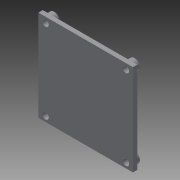
# Autodesk Inventor part: platnickapoddriver
Saved by Autodesk Inventor 2013 (Build 170138000, 138)
## iProperties
Created: 2015-06-20
Part Number: platnickapoddriver
Material: Generic
Document SubType Name: Modeling
Designer: Jufo
Density: 1 g/cm^3
Author: Jufo
Autodesk Inventor part; units mm, degrees
ref_plane "YZ Plane" through (0, 0, 0) normal (1, 0, 0) x (0, 1, 0)
ref_plane "XZ Plane" through (0, 0, 0) normal (0, 1, 0) x (-1, 0, 0)
ref_plane "XY Plane" through (0, 0, 0) normal (0, 0, 1) x (1, 0, 0)
sketch "Sketch1" plane through (0, 0, 0) normal (0, 1, 0) x (-1, 0, 0)
  line L0 (-19.1238, 18.0952) -> (24.3762, 18.0952)
  line L1 (24.3762, 18.0952) -> (24.3762, -23.9048)
  line L2 (24.3762, -23.9048) -> (-19.1238, -23.9048)
  line L3 (-19.1238, -23.9048) -> (-19.1238, 18.0952)
  circle A0 centre (21.1262, -21.4048) radius 1.5
  circle A1 centre (-15.8738, -21.4048) radius 1.5
  line L4 (25.2561, -2.9048) -> (4.7067, -2.9048)
  circle A2 centre (21.1262, 15.5952) radius 1.5
  circle A3 centre (-15.8738, 15.5952) radius 1.5
  point P0 (0, 0)
  dimension "d0" = 43.5
  dimension "d2" = 42
  dimension "d3" = 3
  dimension "d4" = 3
  dimension "d7" = 3.25
  dimension "d8" = 2.5
  dimension "d9" = 3.25
  dimension "d10" = 2.5
  constraints: 10 end point, 4 centre point, 2 parallel, 2 perpendicular, 2 symmetric about line, 1 horizontal, 2 other
  measures "d0" distance of L1.end L2.end
  measures "d2" distance of L0.end L1.end
  measures "d3" diameter of A0
  measures "d4" diameter of A1
  measures "d7" distance from line of L3 A1.centre
  measures "d8" distance from line of L2 A1.centre
  measures "d9" distance from line of L1 A0.centre
  measures "d10" distance from line of L2 A0.centre
extrude "Extrusion1" add sketch "Sketch1" along normal blind 2
sketch "Sketch2" plane through (0, 2, 0) normal (0, 1, 0) x (1, 0, 0)
  circle A0 centre (-21.1262, -15.5952) radius 1.5 projected
  circle A1 centre (15.8738, -15.5952) radius 1.5 projected
  circle A2 centre (15.8738, 21.4048) radius 1.5 projected
  circle A3 centre (-21.1262, 21.4048) radius 1.5 projected
  circle A4 centre (-21.1262, -15.5952) radius 2.5
  circle A5 centre (15.8738, -15.5952) radius 2.5
  circle A6 centre (15.8738, 21.4048) radius 2.5
  circle A7 centre (-21.1262, 21.4048) radius 2.5
  point P0 (0, 0)
  dimension "d13" = 5
  dimension "d14" = 5
  constraints: 4 centre point, 4 coincident
  measures "d13" diameter of A4
  measures "d14" diameter of A5
extrude "Extrusion2" add sketch "Sketch2" along normal blind 2
body "Solid1"
